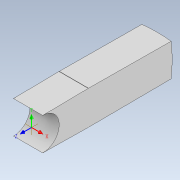
# Autodesk Inventor part: shank_inventor
Saved by Autodesk Inventor 2020 (Build 240168000, 168)
## iProperties
Created: 2021-01-07
Part Number: shank_inventor
Material: Generic
Document SubType Name: Modeling
Designer: DELL
Density: 1 g/cm^3
Appearance: Default
Author: DELL
Autodesk Inventor part; units mm, degrees
ref_plane "YZ Plane" through (0, 0, 0) normal (1, 0, 0) x (0, 1, 0)
ref_plane "XY Plane" through (0, 0, 0) normal (0, 0, 1) x (1, 0, 0)
ref_plane "UCS1: YZ Plane" through (0, 0, 0) normal (1, 0, 0) x (0, 1, 0)
sketch "Sketch2" plane through (0, 0, 0) normal (1, 0, 0) x (0, 1, 0)
  circle A0 centre (0, -70) radius 26
  line L0 (25, -200) -> (-25, -200)
  line L1 (0, -70) -> (0, -200) construction
  line L2 (-25.9992, -70.2001) -> (-25, -200)
  line L3 (25.9992, -70.2001) -> (25, -200)
  circle A1 centre (0, 0) radius 25
  line L4 (-24.9974, 0.3571) -> (-25.9973, -69.6286)
  line L5 (24.9974, 0.3571) -> (25.9973, -69.6286)
  point P0 (25, 0)
  point P1 (-25, 0)
  dimension "d1" = 52
  dimension "d3" = 50
  dimension "d25" = 130
  dimension "d26" = 50
  dimension "d33" = 70
  constraints: 12 end point, 8 point on circle, 5 tangent, 2 centre point, 1 coincident, 1 horizontal, 1 midpoint, 1 perpendicular, 1 vertical alignment, 1 other
  measures "d1" diameter of A0
  measures "d3" distance of L0.start L0.end
  measures "d25" distance from line of L0 L1.start
  measures "d26" diameter of A1
  measures "d33" distance of L1.start A1.centre
extrude "Extrusion1" add sketch "Sketch2" along normal blind 17.5 and the other way blind 27.5 contours A0
extrude "Extrusion2" add sketch "Sketch2" against normal blind 45 from surface at 17.5 contours L3 L0 L2 A0
sketch "Sketch5" plane through (17.5, -25, -200) normal (0, 0, -1) x (-1, 0, 0)
  circle A0 centre (22.5, 25) radius 10
  line L0 (45, 50) -> (45, 0) projected
  line L1 (45, 50) -> (0, 50) projected
  point P0 (17.5, 25)
  point P1 (45, 25)
  point P2 (-45, 0)
  point P3 (22.5, 50)
  dimension "d22" = 20
  constraints: 1 centre point, 1 horizontal alignment, 1 midpoint, 1 vertical alignment, 2 other
  measures "d22" diameter of A0
extrude "Extrusion4" cut sketch "Sketch5" against normal blind 60
ref_plane "Work Plane1" through (-5, 0, -70) normal (-1, 0, 0) x (0, 0, -1)
sketch "Sketch4" plane through (-5, 0, -70) normal (-1, 0, 0) x (0, 0, -1)
  circle A0 centre (-70, 0) radius 200
  line L0 (130, -25) -> (130, 25) projected
  line L1 (-270, 0) -> (130, 0)
  line L2 (130, 0) -> (130, 25)
  line L3 (130, 25) -> (0.2001, 25.9992) projected
  line L4 (130, 25) -> (130.19, 49.679)
  line L5 (130.19, 49.679) -> (123.719, 49.7288)
  point P0 (128.4298, 25.0121)
  point P1 (130, 0)
  constraints: 8 end point, 2 midpoint, 2 perpendicular, 2 point on circle, 1 centre point, 1 coincident, 1 tangent, 1 vertical
revolve "Revolution1" cut sketch "Sketch4" angle 360 about axis through (-5, 0, 200) along (0, 0, -1) contours L5 L4 L3 A0 | L3 L0 A0
extrude "Extrusion5" add sketch "Sketch2" along normal blind 17.5 and the other way blind 27.5 contours A0 L4 A1 L5
body "Solid1"
